Autodesk Inventor part; units mm, degrees
(part 2 of 3)
sketch "Эскиз4" plane through (0, 2, 0) normal (0, 1, 0) x (1, 0, 0)
  arc A0 (90.4395, -37.7453) -> (97.9653, -2.6059) centre (0, 0) ccw construction
  arc A1 (87.1795, -38.3892) -> (90.4395, -37.7453) centre (88.5938, -36.975) ccw construction
  line L0 (87.1795, -38.3892) -> (83.085, -34.2947) construction
  arc A2 (83.085, -34.2947) -> (76.014, -34.2947) centre (79.5495, -37.8302) ccw construction
  line L1 (76.014, -34.2947) -> (67.8823, -42.4264) construction
  line L2 (67.8823, -42.4264) -> (47.1257, -21.6698) construction
  arc A3 (47.1257, -21.6698) -> (46.1335, -19.2746) centre (43.1335, -21.9203) ccw construction
  line L3 (46.1335, -19.2746) -> (46.1335, 19.2746) construction
  arc A4 (46.1335, 19.2746) -> (47.1257, 21.6698) centre (43.1335, 21.9203) ccw construction
  line L4 (47.1257, 21.6698) -> (67.8823, 42.4264) construction
  line L5 (67.8823, 42.4264) -> (76.014, 34.2947) construction
  arc A5 (76.014, 34.2947) -> (83.085, 34.2947) centre (79.5495, 37.8302) ccw construction
  line L6 (83.085, 34.2947) -> (87.1795, 38.3892) construction
  arc A6 (90.4395, 37.7453) -> (87.1795, 38.3892) centre (88.5938, 36.975) ccw construction
  arc A7 (97.9653, 2.6059) -> (90.4395, 37.7453) centre (0, 0) ccw construction
  arc A8 (97.9653, 2.6059) -> (97.9653, -2.6059) centre (101, 0) ccw construction
  circle A9 centre (101, 0) radius 1.9 construction
  arc A10 (93.0503, -48.6481) -> (93.0503, 48.6481) centre (0, 0) ccw construction
  arc A11 (93.0503, 48.6481) -> (88.2704, 49.3795) centre (90.3917, 47.2582) ccw construction
  line L7 (88.2704, 49.3795) -> (85.2064, 46.3155) construction
  arc A12 (73.8927, 46.3155) -> (85.2064, 46.3155) centre (79.5495, 51.9723) ccw construction
  line L8 (73.8927, 46.3155) -> (46.3155, 73.8927) construction
  arc A13 (46.3155, 85.2064) -> (46.3155, 73.8927) centre (51.9723, 79.5495) ccw construction
  line L9 (46.3155, 85.2064) -> (49.3795, 88.2704) construction
  arc A14 (49.3795, 88.2704) -> (48.6481, 93.0503) centre (47.2582, 90.3917) ccw construction
  arc A15 (48.6481, 93.0503) -> (-48.6481, 93.0503) centre (0, 0) ccw construction
  arc A16 (-48.6481, 93.0503) -> (-49.3795, 88.2704) centre (-47.2582, 90.3917) ccw construction
  line L10 (-49.3795, 88.2704) -> (-46.3155, 85.2064) construction
  arc A17 (-46.3155, 73.8927) -> (-46.3155, 85.2064) centre (-51.9723, 79.5495) ccw construction
  line L11 (-46.3155, 73.8927) -> (-73.8927, 46.3155) construction
  arc A18 (-85.2064, 46.3155) -> (-73.8927, 46.3155) centre (-79.5495, 51.9723) ccw construction
  line L12 (-85.2064, 46.3155) -> (-88.2704, 49.3795) construction
  arc A19 (-88.2704, 49.3795) -> (-93.0503, 48.6481) centre (-90.3917, 47.2582) ccw construction
  arc A20 (-93.0503, 48.6481) -> (-93.0503, -48.6481) centre (0, 0) ccw construction
  arc A21 (-93.0503, -48.6481) -> (-88.2704, -49.3795) centre (-90.3917, -47.2582) ccw construction
  line L13 (-88.2704, -49.3795) -> (-85.2064, -46.3155) construction
  arc A22 (-73.8927, -46.3155) -> (-85.2064, -46.3155) centre (-79.5495, -51.9723) ccw construction
  line L14 (-73.8927, -46.3155) -> (-46.3155, -73.8927) construction
  arc A23 (-46.3155, -85.2064) -> (-46.3155, -73.8927) centre (-51.9723, -79.5495) ccw construction
  line L15 (-46.3155, -85.2064) -> (-49.3795, -88.2704) construction
  arc A24 (-49.3795, -88.2704) -> (-48.6481, -93.0503) centre (-47.2582, -90.3917) ccw construction
  arc A25 (-48.6481, -93.0503) -> (-45.42, -94.668) centre (0, 0) ccw construction
  arc A26 (-45.42, -94.668) -> (-43.0355, -94.1655) centre (-44.5548, -92.8648) ccw construction
  line L16 (-43.0355, -94.1655) -> (-18.3802, -65.3664) construction
  arc A27 (-17.477, -64.7643) -> (-18.3802, -65.3664) centre (-16.8609, -66.6671) ccw construction
  line L17 (-17.477, -64.7643) -> (-0.6161, -59.3045) construction
  arc A28 (0.6161, -59.3045) -> (-0.6161, -59.3045) centre (0, -61.2072) ccw construction
  line L18 (0.6161, -59.3045) -> (17.477, -64.7643) construction
  arc A29 (18.3802, -65.3664) -> (17.477, -64.7643) centre (16.8609, -66.6671) ccw construction
  line L19 (18.3802, -65.3664) -> (43.0355, -94.1655) construction
  arc A30 (43.0355, -94.1655) -> (45.42, -94.668) centre (44.5548, -92.8648) ccw construction
  arc A31 (45.42, -94.668) -> (48.6481, -93.0503) centre (0, 0) ccw construction
  arc A32 (48.6481, -93.0503) -> (49.3795, -88.2704) centre (47.2582, -90.3917) ccw construction
  line L20 (49.3795, -88.2704) -> (46.3155, -85.2064) construction
  arc A33 (46.3155, -73.8927) -> (46.3155, -85.2064) centre (51.9723, -79.5495) ccw construction
  line L21 (46.3155, -73.8927) -> (73.8927, -46.3155) construction
  arc A34 (85.2064, -46.3155) -> (73.8927, -46.3155) centre (79.5495, -51.9723) ccw construction
  line L22 (85.2064, -46.3155) -> (88.2704, -49.3795) construction
  arc A35 (88.2704, -49.3795) -> (93.0503, -48.6481) centre (90.3917, -47.2582) ccw construction
  circle A36 centre (-101, 0) radius 1.9 construction
  arc A37 (-90.4395, 37.7453) -> (-97.9653, 2.6059) centre (0, 0) ccw construction
  arc A38 (-87.1795, 38.3892) -> (-90.4395, 37.7453) centre (-88.5938, 36.975) ccw construction
  line L23 (-87.1795, 38.3892) -> (-83.085, 34.2947) construction
  arc A39 (-83.085, 34.2947) -> (-76.014, 34.2947) centre (-79.5495, 37.8302) ccw construction
  line L24 (-76.014, 34.2947) -> (-67.8823, 42.4264) construction
  line L25 (-67.8823, 42.4264) -> (-47.1257, 21.6698) construction
  arc A40 (-47.1257, 21.6698) -> (-46.1335, 19.2746) centre (-43.1335, 21.9203) ccw construction
  line L26 (-46.1335, 19.2746) -> (-46.1335, -19.2746) construction
  arc A41 (-46.1335, -19.2746) -> (-47.1257, -21.6698) centre (-43.1335, -21.9203) ccw construction
  line L27 (-47.1257, -21.6698) -> (-67.8823, -42.4264) construction
  line L28 (-67.8823, -42.4264) -> (-76.014, -34.2947) construction
  arc A42 (-76.014, -34.2947) -> (-83.085, -34.2947) centre (-79.5495, -37.8302) ccw construction
  line L29 (-83.085, -34.2947) -> (-87.1795, -38.3892) construction
  arc A43 (-90.4395, -37.7453) -> (-87.1795, -38.3892) centre (-88.5938, -36.975) ccw construction
  arc A44 (-97.9653, -2.6059) -> (-90.4395, -37.7453) centre (0, 0) ccw construction
  arc A45 (-97.9653, -2.6059) -> (-97.9653, 2.6059) centre (-101, 0) ccw construction
  circle A46 centre (45.1111, -90.3659) radius 2 construction
  circle A47 centre (45.1111, 90.3659) radius 2 construction
  circle A48 centre (90.3659, 45.1111) radius 2 construction
  circle A49 centre (-45.1111, -90.3659) radius 2 construction
  circle A50 centre (90.3659, -45.1111) radius 2 construction
  circle A51 centre (-45.1111, 90.3659) radius 2 construction
  circle A52 centre (-90.3659, 45.1111) radius 2 construction
  circle A53 centre (-90.3659, -45.1111) radius 2 construction
  line L30 (-63.6396, -46.669) -> (-43.8406, -26.8701) construction
  arc A54 (-41.0122, -26.8701) -> (-43.8406, -26.8701) centre (-42.4264, -28.2843) ccw construction
  line L31 (-41.0122, -26.8701) -> (-26.8701, -41.0122) construction
  arc A55 (-26.8701, -43.8406) -> (-26.8701, -41.0122) centre (-28.2843, -42.4264) ccw construction
  line L32 (-26.8701, -43.8406) -> (-46.669, -63.6396) construction
  line L33 (-46.669, -63.6396) -> (-63.6396, -46.669) construction
  line L34 (-42.4264, -67.8823) -> (-21.6698, -47.1257) construction
  arc A56 (-21.6698, -47.1257) -> (-19.2746, -46.1335) centre (-21.9203, -43.1335) ccw construction
  line L35 (-19.2746, -46.1335) -> (19.2746, -46.1335) construction
  arc A57 (19.2746, -46.1335) -> (21.6698, -47.1257) centre (21.9203, -43.1335) ccw construction
  line L36 (21.6698, -47.1257) -> (42.4264, -67.8823) construction
  line L37 (42.4264, -67.8823) -> (37.1244, -73.1843) construction
  arc A58 (34.1909, -73.0707) -> (37.1244, -73.1843) centre (35.7102, -71.7701) ccw construction
  line L38 (34.1909, -73.0707) -> (25.4187, -62.8242) construction
  arc A59 (24.842, -61.8893) -> (25.4187, -62.8242) centre (28.1154, -60.5155) ccw construction
  line L39 (24.842, -61.8893) -> (23.8313, -59.4808) construction
  arc A60 (23.8313, -59.4808) -> (21.0049, -57.3328) centre (20.5578, -60.8546) ccw construction
  line L40 (21.0049, -57.3328) -> (15.1585, -56.5907) construction
  arc A61 (14.5119, -56.4463) -> (15.1585, -56.5907) centre (15.6055, -53.069) ccw construction
  line L41 (14.5119, -56.4463) -> (0.6161, -51.9466) construction
  arc A62 (0.6161, -51.9466) -> (-0.6161, -51.9466) centre (0, -53.8493) ccw construction
  line L42 (-0.6161, -51.9466) -> (-14.5119, -56.4463) construction
  arc A63 (-15.1585, -56.5907) -> (-14.5119, -56.4463) centre (-15.6055, -53.069) ccw construction
  line L43 (-15.1585, -56.5907) -> (-21.0049, -57.3328) construction
  arc A64 (-21.0049, -57.3328) -> (-23.8313, -59.4808) centre (-20.5578, -60.8546) ccw construction
  line L44 (-23.8313, -59.4808) -> (-24.842, -61.8893) construction
  arc A65 (-25.4187, -62.8242) -> (-24.842, -61.8893) centre (-28.1154, -60.5155) ccw construction
  line L45 (-25.4187, -62.8242) -> (-34.1909, -73.0707) construction
  arc A66 (-37.1244, -73.1843) -> (-34.1909, -73.0707) centre (-35.7102, -71.7701) ccw construction
  line L46 (-37.1244, -73.1843) -> (-42.4264, -67.8823) construction
  line L47 (46.669, -63.6396) -> (26.8701, -43.8406) construction
  arc A67 (26.8701, -41.0122) -> (26.8701, -43.8406) centre (28.2843, -42.4264) ccw construction
  line L48 (26.8701, -41.0122) -> (41.0122, -26.8701) construction
  arc A68 (43.8406, -26.8701) -> (41.0122, -26.8701) centre (42.4264, -28.2843) ccw construction
  line L49 (43.8406, -26.8701) -> (63.6396, -46.669) construction
  line L50 (63.6396, -46.669) -> (46.669, -63.6396) construction
  line L51 (63.6396, 46.669) -> (43.8406, 26.8701) construction
  arc A69 (41.0122, 26.8701) -> (43.8406, 26.8701) centre (42.4264, 28.2843) ccw construction
  line L52 (41.0122, 26.8701) -> (26.8701, 41.0122) construction
  arc A70 (26.8701, 43.8406) -> (26.8701, 41.0122) centre (28.2843, 42.4264) ccw construction
  line L53 (26.8701, 43.8406) -> (46.669, 63.6396) construction
  line L54 (46.669, 63.6396) -> (63.6396, 46.669) construction
  line L55 (42.4264, 67.8823) -> (21.6698, 47.1257) construction
  arc A71 (21.6698, 47.1257) -> (19.2746, 46.1335) centre (21.9203, 43.1335) ccw construction
  line L56 (19.2746, 46.1335) -> (-19.2746, 46.1335) construction
  arc A72 (-19.2746, 46.1335) -> (-21.6698, 47.1257) centre (-21.9203, 43.1335) ccw construction
  line L57 (-21.6698, 47.1257) -> (-42.4264, 67.8823) construction
  line L58 (-42.4264, 67.8823) -> (-34.2947, 76.014) construction
  arc A73 (-34.2947, 76.014) -> (-34.2947, 83.085) centre (-37.8302, 79.5495) ccw construction
  line L59 (-34.2947, 83.085) -> (-38.3892, 87.1795) construction
  arc A74 (-37.7453, 90.4395) -> (-38.3892, 87.1795) centre (-36.975, 88.5938) ccw construction
  arc A75 (37.7453, 90.4395) -> (-37.7453, 90.4395) centre (0, 0) ccw construction
  arc A76 (38.3892, 87.1795) -> (37.7453, 90.4395) centre (36.975, 88.5938) ccw construction
  line L60 (38.3892, 87.1795) -> (34.2947, 83.085) construction
  arc A77 (34.2947, 83.085) -> (34.2947, 76.014) centre (37.8302, 79.5495) ccw construction
  line L61 (34.2947, 76.014) -> (42.4264, 67.8823) construction
  line L62 (-19.2746, 40.1335) -> (19.2746, 40.1335) construction
  arc A78 (19.2746, 40.1335) -> (21.6698, 39.1414) centre (21.9203, 43.1335) ccw construction
  line L63 (21.6698, 39.1414) -> (39.1414, 21.6698) construction
  arc A79 (39.1414, 21.6698) -> (40.1335, 19.2746) centre (43.1335, 21.9203) ccw construction
  line L64 (40.1335, 19.2746) -> (40.1335, -19.2746) construction
  arc A80 (40.1335, -19.2746) -> (39.1414, -21.6698) centre (43.1335, -21.9203) ccw construction
  line L65 (39.1414, -21.6698) -> (21.6698, -39.1414) construction
  arc A81 (21.6698, -39.1414) -> (19.2746, -40.1335) centre (21.9203, -43.1335) ccw construction
  line L66 (19.2746, -40.1335) -> (-19.2746, -40.1335) construction
  arc A82 (-19.2746, -40.1335) -> (-21.6698, -39.1414) centre (-21.9203, -43.1335) ccw construction
  line L67 (-21.6698, -39.1414) -> (-39.1414, -21.6698) construction
  arc A83 (-39.1414, -21.6698) -> (-40.1335, -19.2746) centre (-43.1335, -21.9203) ccw construction
  line L68 (-40.1335, -19.2746) -> (-40.1335, 19.2746) construction
  arc A84 (-40.1335, 19.2746) -> (-39.1414, 21.6698) centre (-43.1335, 21.9203) ccw construction
  line L69 (-39.1414, 21.6698) -> (-21.6698, 39.1414) construction
  arc A85 (-21.6698, 39.1414) -> (-19.2746, 40.1335) centre (-21.9203, 43.1335) ccw construction
  circle A86 centre (43.1335, 21.9203) radius 1.6 construction
  circle A87 centre (21.9203, -43.1335) radius 1.6 construction
  circle A88 centre (-21.9203, -43.1335) radius 1.6 construction
  circle A89 centre (-43.1335, -21.9203) radius 1.6 construction
  circle A90 centre (-43.1335, 21.9203) radius 1.6 construction
  circle A91 centre (-21.9203, 43.1335) radius 1.6 construction
  circle A92 centre (43.1335, -21.9203) radius 1.6 construction
  circle A93 centre (21.9203, 43.1335) radius 1.6 construction
  circle A94 centre (-37.8302, 79.5495) radius 1.6 construction
  circle A95 centre (-79.5495, 37.8302) radius 1.6 construction
  circle A96 centre (-79.5495, -37.8302) radius 1.6 construction
  circle A97 centre (79.5495, -37.8302) radius 1.6 construction
  circle A98 centre (37.8302, 79.5495) radius 1.6 construction
  circle A99 centre (79.5495, 37.8302) radius 1.6 construction
  circle A100 centre (-20.5578, -60.8546) radius 1.55 construction
  circle A101 centre (20.5578, -60.8546) radius 1.55 construction
  circle A102 centre (37.8302, -79.5495) radius 1.6 construction
  circle A103 centre (-37.8302, -79.5495) radius 1.6 construction
  line L70 (-46.669, 63.6396) -> (-26.8701, 43.8406) construction
  arc A104 (-26.8701, 41.0122) -> (-26.8701, 43.8406) centre (-28.2843, 42.4264) ccw construction
  line L71 (-26.8701, 41.0122) -> (-41.0122, 26.8701) construction
  arc A105 (-43.8406, 26.8701) -> (-41.0122, 26.8701) centre (-42.4264, 28.2843) ccw construction
  line L72 (-43.8406, 26.8701) -> (-63.6396, 46.669) construction
  line L73 (-63.6396, 46.669) -> (-46.669, 63.6396) construction
  circle A106 centre (0, 0) radius 101 construction
  circle A107 centre (-24, 98.1071) radius 1.6
  circle A108 centre (-24, 98.1071) radius 4
  line L74 (19.2746, 46.1335) -> (-19.2746, 46.1335) construction
  line L75 (0, 46.1335) -> (0, 40.1335) construction
  circle A109 centre (0, 46) radius 1.6
  arc A110 (-3.9978, 46.1335) -> (3.9978, 46.1335) centre (0, 46) ccw construction
  line L76 (-19.2746, 46.1335) -> (-6.2595, 46.1335) construction
  line L77 (6.2595, 46.1335) -> (19.2746, 46.1335) construction
  arc A111 (3.5768, 47.7906) -> (-3.5768, 47.7906) centre (0, 46) ccw
  arc A112 (-6.2595, 46.1335) -> (-3.5768, 47.7906) centre (-6.2595, 49.1335) ccw
  arc A113 (3.5768, 47.7906) -> (6.2595, 46.1335) centre (6.2595, 49.1335) ccw
  line L78 (6.2595, 46.1335) -> (6.2595, 42.1115)
  line L79 (6.2595, 42.1115) -> (-6.2595, 42.1115)
  line L80 (-6.2595, 42.1115) -> (-6.2595, 46.1335)
  line L81 (0, 0) -> (-30.4056, 30.4056) construction
  line L82 (-46.1335, -19.2746) -> (-46.1335, 19.2746) construction
  line L83 (-46.1335, -19.2746) -> (-46.1335, 19.2746) construction
  line L84 (-46.1335, 0) -> (-40.1335, 0) construction
  circle A114 centre (-46, 0) radius 1.6
  arc A115 (-46.1335, -3.9978) -> (-46.1335, 3.9978) centre (-46, 0) ccw construction
  line L85 (-46.1335, 19.2746) -> (-46.1335, 6.2595) construction
  line L86 (-46.1335, -6.2595) -> (-46.1335, -19.2746) construction
  arc A116 (-47.7906, 3.5768) -> (-47.7906, -3.5768) centre (-46, 0) ccw
  arc A117 (-47.7906, 3.5768) -> (-46.1335, 6.2595) centre (-49.1335, 6.2595) ccw
  arc A118 (-46.1335, -6.2595) -> (-47.7906, -3.5768) centre (-49.1335, -6.2595) ccw
  line L87 (-46.1335, -6.2595) -> (-42.1115, -6.2595)
  line L88 (-42.1115, -6.2595) -> (-42.1115, 6.2595)
  line L89 (-42.1115, 6.2595) -> (-46.1335, 6.2595)
  line L90 (0, 0) -> (0, -40.1335) construction
  line L91 (42.1115, 6.2595) -> (46.1335, 6.2595)
  line L92 (42.1115, -6.2595) -> (42.1115, 6.2595)
  arc A119 (46.1335, 6.2595) -> (47.7906, 3.5768) centre (49.1335, 6.2595) ccw
  arc A120 (47.7906, -3.5768) -> (47.7906, 3.5768) centre (46, 0) ccw
  arc A121 (47.7906, -3.5768) -> (46.1335, -6.2595) centre (49.1335, -6.2595) ccw
  line L93 (46.1335, -6.2595) -> (42.1115, -6.2595)
  circle A122 centre (46, 0) radius 1.6
  arc A123 (46.1335, 3.9978) -> (46.1335, -3.9978) centre (46, 0) ccw construction
  circle A124 centre (24, 98.1071) radius 1.6
  circle A125 centre (24, 98.1071) radius 4
  point P0 (46.1335, 0)
  point P1 (0, 101)
  dimension "d89" = 202
  dimension "d90" = 3.2
  dimension "d91" = 8
  dimension "d92" = 3.2
  dimension "d94" = 8
  dimension "d95" = 3
  dimension "d109" = 55
  dimension "d110" = 48
  constraints: 38 end point, 32 point on circle, 29 symmetric about line, 20 centre point, 11 point on line, 6 coincident, 4 midpoint, 4 tangent, 2 perpendicular, 1 collinear, 1 equal radius, 1 vertical, 12 other
  measures "d89" diameter of A106
  measures "d90" diameter of A107
  measures "d91" diameter of A108
  measures "d92" diameter of A109
  measures "d94" diameter of A110
  measures "d95" radius of A112
  measures "d109" distance of A106.end A109.centre
  measures "d110" distance of A124.centre A107.centre
extrude "Выдавливание5" cut sketch "Эскиз4" against normal blind 2 contours A107 | A109 | A114 | A122 | A124
extrude "Выдавливание6" add sketch "Эскиз4" against normal blind 2
sketch "Эскиз5" plane through (0, 2, 0) normal (0, 1, 0) x (1, 0, 0)
  circle A0 centre (-46, 0) radius 1.6 construction
  line L0 (-6.2595, 46.1335) -> (-19.2746, 46.1335) construction
  arc A1 (-19.2746, 46.1335) -> (-21.6698, 47.1257) centre (-21.9203, 43.1335) ccw construction
  line L1 (-21.6698, 47.1257) -> (-42.4264, 67.8823) construction
  line L2 (-42.4264, 67.8823) -> (-34.2947, 76.014) construction
  arc A2 (-34.2947, 76.014) -> (-34.2947, 83.085) centre (-37.8302, 79.5495) ccw construction
  line L3 (-34.2947, 83.085) -> (-38.3892, 87.1795) construction
  arc A3 (-37.7453, 90.4395) -> (-38.3892, 87.1795) centre (-36.975, 88.5938) ccw construction
  arc A4 (-25.8102, 94.5401) -> (-37.7453, 90.4395) centre (0, 0) ccw construction
  arc A5 (-25.8102, 94.5401) -> (-20.7476, 95.7786) centre (-24, 98.1071) ccw construction
  arc A6 (20.7476, 95.7786) -> (-20.7476, 95.7786) centre (0, 0) ccw construction
  arc A7 (38.3892, 87.1795) -> (37.7453, 90.4395) centre (36.975, 88.5938) ccw construction
  line L4 (38.3892, 87.1795) -> (34.2947, 83.085) construction
  arc A8 (34.2947, 83.085) -> (34.2947, 76.014) centre (37.8302, 79.5495) ccw construction
  line L5 (34.2947, 76.014) -> (42.4264, 67.8823) construction
  line L6 (42.4264, 67.8823) -> (21.6698, 47.1257) construction
  arc A9 (21.6698, 47.1257) -> (19.2746, 46.1335) centre (21.9203, 43.1335) ccw construction
  line L7 (19.2746, 46.1335) -> (6.2595, 46.1335) construction
  arc A10 (3.5768, 47.7906) -> (6.2595, 46.1335) centre (6.2595, 49.1335) ccw construction
  arc A11 (3.5768, 47.7906) -> (-3.5768, 47.7906) centre (0, 46) ccw construction
  arc A12 (-6.2595, 46.1335) -> (-3.5768, 47.7906) centre (-6.2595, 49.1335) ccw construction
  circle A13 centre (46, 0) radius 1.6 construction
  arc A14 (48.6481, 93.0503) -> (-48.6481, 93.0503) centre (0, 0) ccw construction
  arc A15 (-48.6481, 93.0503) -> (-49.3795, 88.2704) centre (-47.2582, 90.3917) ccw construction
  line L8 (-49.3795, 88.2704) -> (-46.3155, 85.2064) construction
  arc A16 (-46.3155, 73.8927) -> (-46.3155, 85.2064) centre (-51.9723, 79.5495) ccw construction
  line L9 (-46.3155, 73.8927) -> (-73.8927, 46.3155) construction
  arc A17 (-85.2064, 46.3155) -> (-73.8927, 46.3155) centre (-79.5495, 51.9723) ccw construction
  line L10 (-85.2064, 46.3155) -> (-88.2704, 49.3795) construction
  arc A18 (-88.2704, 49.3795) -> (-93.0503, 48.6481) centre (-90.3917, 47.2582) ccw construction
  arc A19 (-93.0503, 48.6481) -> (-93.0503, -48.6481) centre (0, 0) ccw construction
  arc A20 (-93.0503, -48.6481) -> (-88.2704, -49.3795) centre (-90.3917, -47.2582) ccw construction
  line L11 (-88.2704, -49.3795) -> (-85.2064, -46.3155) construction
  arc A21 (-73.8927, -46.3155) -> (-85.2064, -46.3155) centre (-79.5495, -51.9723) ccw construction
  line L12 (-73.8927, -46.3155) -> (-46.3155, -73.8927) construction
  arc A22 (-46.3155, -85.2064) -> (-46.3155, -73.8927) centre (-51.9723, -79.5495) ccw construction
  line L13 (-46.3155, -85.2064) -> (-49.3795, -88.2704) construction
  arc A23 (-49.3795, -88.2704) -> (-48.6481, -93.0503) centre (-47.2582, -90.3917) ccw construction
  arc A24 (-48.6481, -93.0503) -> (-45.42, -94.668) centre (0, 0) ccw construction
  arc A25 (-45.42, -94.668) -> (-43.0355, -94.1655) centre (-44.5548, -92.8648) ccw construction
  line L14 (-43.0355, -94.1655) -> (-18.3802, -65.3664) construction
  arc A26 (-17.477, -64.7643) -> (-18.3802, -65.3664) centre (-16.8609, -66.6671) ccw construction
  line L15 (-17.477, -64.7643) -> (-0.6161, -59.3045) construction
  arc A27 (0.6161, -59.3045) -> (-0.6161, -59.3045) centre (0, -61.2072) ccw construction
  line L16 (0.6161, -59.3045) -> (17.477, -64.7643) construction
  arc A28 (18.3802, -65.3664) -> (17.477, -64.7643) centre (16.8609, -66.6671) ccw construction
  line L17 (18.3802, -65.3664) -> (43.0355, -94.1655) construction
  arc A29 (43.0355, -94.1655) -> (45.42, -94.668) centre (44.5548, -92.8648) ccw construction
  arc A30 (45.42, -94.668) -> (48.6481, -93.0503) centre (0, 0) ccw construction
  arc A31 (48.6481, -93.0503) -> (49.3795, -88.2704) centre (47.2582, -90.3917) ccw construction
  line L18 (49.3795, -88.2704) -> (46.3155, -85.2064) construction
  arc A32 (46.3155, -73.8927) -> (46.3155, -85.2064) centre (51.9723, -79.5495) ccw construction
  line L19 (46.3155, -73.8927) -> (73.8927, -46.3155) construction
  arc A33 (85.2064, -46.3155) -> (73.8927, -46.3155) centre (79.5495, -51.9723) ccw construction
  line L20 (85.2064, -46.3155) -> (88.2704, -49.3795) construction
  arc A34 (88.2704, -49.3795) -> (93.0503, -48.6481) centre (90.3917, -47.2582) ccw construction
  arc A35 (93.0503, -48.6481) -> (93.0503, 48.6481) centre (0, 0) ccw construction
  arc A36 (93.0503, 48.6481) -> (88.2704, 49.3795) centre (90.3917, 47.2582) ccw construction
  line L21 (88.2704, 49.3795) -> (85.2064, 46.3155) construction
  arc A37 (73.8927, 46.3155) -> (85.2064, 46.3155) centre (79.5495, 51.9723) ccw construction
  line L22 (73.8927, 46.3155) -> (46.3155, 73.8927) construction
  arc A38 (46.3155, 85.2064) -> (46.3155, 73.8927) centre (51.9723, 79.5495) ccw construction
  line L23 (46.3155, 85.2064) -> (49.3795, 88.2704) construction
  arc A39 (49.3795, 88.2704) -> (48.6481, 93.0503) centre (47.2582, 90.3917) ccw construction
  circle A40 centre (-24, 98.1071) radius 1.6 construction
  circle A41 centre (0, 46) radius 1.6 construction
  arc A42 (47.7906, -3.5768) -> (46.1335, -6.2595) centre (49.1335, -6.2595) ccw construction
  arc A43 (47.7906, -3.5768) -> (47.7906, 3.5768) centre (46, 0) ccw construction
  arc A44 (46.1335, 6.2595) -> (47.7906, 3.5768) centre (49.1335, 6.2595) ccw construction
  line L24 (46.1335, 6.2595) -> (46.1335, 19.2746) construction
  arc A45 (46.1335, 19.2746) -> (47.1257, 21.6698) centre (43.1335, 21.9203) ccw construction
  line L25 (47.1257, 21.6698) -> (67.8823, 42.4264) construction
  line L26 (67.8823, 42.4264) -> (76.014, 34.2947) construction
  arc A46 (76.014, 34.2947) -> (83.085, 34.2947) centre (79.5495, 37.8302) ccw construction
  line L27 (83.085, 34.2947) -> (87.1795, 38.3892) construction
  arc A47 (90.4395, 37.7453) -> (87.1795, 38.3892) centre (88.5938, 36.975) ccw construction
  arc A48 (97.9653, 2.6059) -> (90.4395, 37.7453) centre (0, 0) ccw construction
  arc A49 (97.9653, 2.6059) -> (97.9653, -2.6059) centre (101, 0) ccw construction
  arc A50 (90.4395, -37.7453) -> (97.9653, -2.6059) centre (0, 0) ccw construction
  arc A51 (87.1795, -38.3892) -> (90.4395, -37.7453) centre (88.5938, -36.975) ccw construction
  line L28 (87.1795, -38.3892) -> (83.085, -34.2947) construction
  arc A52 (83.085, -34.2947) -> (76.014, -34.2947) centre (79.5495, -37.8302) ccw construction
  line L29 (76.014, -34.2947) -> (67.8823, -42.4264) construction
  line L30 (67.8823, -42.4264) -> (47.1257, -21.6698) construction
  arc A53 (47.1257, -21.6698) -> (46.1335, -19.2746) centre (43.1335, -21.9203) ccw construction
  line L31 (46.1335, -19.2746) -> (46.1335, -6.2595) construction
  circle A54 centre (101, 0) radius 1.9 construction
  circle A55 centre (-101, 0) radius 1.9 construction
  arc A56 (-47.7906, 3.5768) -> (-46.1335, 6.2595) centre (-49.1335, 6.2595) ccw construction
  arc A57 (-47.7906, 3.5768) -> (-47.7906, -3.5768) centre (-46, 0) ccw construction
  arc A58 (-46.1335, -6.2595) -> (-47.7906, -3.5768) centre (-49.1335, -6.2595) ccw construction
  line L32 (-46.1335, -6.2595) -> (-46.1335, -19.2746) construction
  arc A59 (-46.1335, -19.2746) -> (-47.1257, -21.6698) centre (-43.1335, -21.9203) ccw construction
  line L33 (-47.1257, -21.6698) -> (-67.8823, -42.4264) construction
  line L34 (-67.8823, -42.4264) -> (-76.014, -34.2947) construction
  arc A60 (-76.014, -34.2947) -> (-83.085, -34.2947) centre (-79.5495, -37.8302) ccw construction
  line L35 (-83.085, -34.2947) -> (-87.1795, -38.3892) construction
  arc A61 (-90.4395, -37.7453) -> (-87.1795, -38.3892) centre (-88.5938, -36.975) ccw construction
  arc A62 (-97.9653, -2.6059) -> (-90.4395, -37.7453) centre (0, 0) ccw construction
  arc A63 (-97.9653, -2.6059) -> (-97.9653, 2.6059) centre (-101, 0) ccw construction
  arc A64 (-90.4395, 37.7453) -> (-97.9653, 2.6059) centre (0, 0) ccw construction
  arc A65 (-87.1795, 38.3892) -> (-90.4395, 37.7453) centre (-88.5938, 36.975) ccw construction
  line L36 (-87.1795, 38.3892) -> (-83.085, 34.2947) construction
  arc A66 (-83.085, 34.2947) -> (-76.014, 34.2947) centre (-79.5495, 37.8302) ccw construction
  line L37 (-76.014, 34.2947) -> (-67.8823, 42.4264) construction
  line L38 (-67.8823, 42.4264) -> (-47.1257, 21.6698) construction
  arc A67 (-47.1257, 21.6698) -> (-46.1335, 19.2746) centre (-43.1335, 21.9203) ccw construction
  line L39 (-46.1335, 19.2746) -> (-46.1335, 6.2595) construction
  circle A68 centre (45.1111, -90.3659) radius 2 construction
  circle A69 centre (45.1111, 90.3659) radius 2 construction
  circle A70 centre (90.3659, 45.1111) radius 2 construction
  circle A71 centre (-45.1111, -90.3659) radius 2 construction
  circle A72 centre (90.3659, -45.1111) radius 2 construction
  circle A73 centre (-45.1111, 90.3659) radius 2 construction
  circle A74 centre (-90.3659, 45.1111) radius 2 construction
  circle A75 centre (-90.3659, -45.1111) radius 2 construction
  line L40 (-63.6396, -46.669) -> (-43.8406, -26.8701) construction
  arc A76 (-41.0122, -26.8701) -> (-43.8406, -26.8701) centre (-42.4264, -28.2843) ccw construction
  line L41 (-41.0122, -26.8701) -> (-26.8701, -41.0122) construction
  arc A77 (-26.8701, -43.8406) -> (-26.8701, -41.0122) centre (-28.2843, -42.4264) ccw construction
  line L42 (-26.8701, -43.8406) -> (-46.669, -63.6396) construction
  line L43 (-46.669, -63.6396) -> (-63.6396, -46.669) construction
  line L44 (-42.4264, -67.8823) -> (-21.6698, -47.1257) construction
  arc A78 (-21.6698, -47.1257) -> (-19.2746, -46.1335) centre (-21.9203, -43.1335) ccw construction
  line L45 (-19.2746, -46.1335) -> (19.2746, -46.1335) construction
  arc A79 (19.2746, -46.1335) -> (21.6698, -47.1257) centre (21.9203, -43.1335) ccw construction
  line L46 (21.6698, -47.1257) -> (42.4264, -67.8823) construction
  line L47 (42.4264, -67.8823) -> (37.1244, -73.1843) construction
  arc A80 (34.1909, -73.0707) -> (37.1244, -73.1843) centre (35.7102, -71.7701) ccw construction
  line L48 (34.1909, -73.0707) -> (25.4187, -62.8242) construction
  arc A81 (24.842, -61.8893) -> (25.4187, -62.8242) centre (28.1154, -60.5155) ccw construction
  line L49 (24.842, -61.8893) -> (23.8313, -59.4808) construction
  arc A82 (23.8313, -59.4808) -> (21.0049, -57.3328) centre (20.5578, -60.8546) ccw construction
  line L50 (21.0049, -57.3328) -> (15.1585, -56.5907) construction
  arc A83 (14.5119, -56.4463) -> (15.1585, -56.5907) centre (15.6055, -53.069) ccw construction
  line L51 (14.5119, -56.4463) -> (0.6161, -51.9466) construction
  arc A84 (0.6161, -51.9466) -> (-0.6161, -51.9466) centre (0, -53.8493) ccw construction
  line L52 (-0.6161, -51.9466) -> (-14.5119, -56.4463) construction
  arc A85 (-15.1585, -56.5907) -> (-14.5119, -56.4463) centre (-15.6055, -53.069) ccw construction
  line L53 (-15.1585, -56.5907) -> (-21.0049, -57.3328) construction
  arc A86 (-21.0049, -57.3328) -> (-23.8313, -59.4808) centre (-20.5578, -60.8546) ccw construction
  line L54 (-23.8313, -59.4808) -> (-24.842, -61.8893) construction
  arc A87 (-25.4187, -62.8242) -> (-24.842, -61.8893) centre (-28.1154, -60.5155) ccw construction
  line L55 (-25.4187, -62.8242) -> (-34.1909, -73.0707) construction
  arc A88 (-37.1244, -73.1843) -> (-34.1909, -73.0707) centre (-35.7102, -71.7701) ccw construction
  line L56 (-37.1244, -73.1843) -> (-42.4264, -67.8823) construction
  line L57 (46.669, -63.6396) -> (26.8701, -43.8406) construction
  arc A89 (26.8701, -41.0122) -> (26.8701, -43.8406) centre (28.2843, -42.4264) ccw construction
  line L58 (26.8701, -41.0122) -> (41.0122, -26.8701) construction
  arc A90 (43.8406, -26.8701) -> (41.0122, -26.8701) centre (42.4264, -28.2843) ccw construction
  line L59 (43.8406, -26.8701) -> (63.6396, -46.669) construction
  line L60 (63.6396, -46.669) -> (46.669, -63.6396) construction
  line L61 (63.6396, 46.669) -> (43.8406, 26.8701) construction
  arc A91 (41.0122, 26.8701) -> (43.8406, 26.8701) centre (42.4264, 28.2843) ccw construction
  line L62 (41.0122, 26.8701) -> (26.8701, 41.0122) construction
  arc A92 (26.8701, 43.8406) -> (26.8701, 41.0122) centre (28.2843, 42.4264) ccw construction
  line L63 (26.8701, 43.8406) -> (46.669, 63.6396) construction
  line L64 (46.669, 63.6396) -> (63.6396, 46.669) construction
  line L65 (-19.2746, 40.1335) -> (19.2746, 40.1335) construction
  arc A93 (19.2746, 40.1335) -> (21.6698, 39.1414) centre (21.9203, 43.1335) ccw construction
  line L66 (21.6698, 39.1414) -> (39.1414, 21.6698) construction
  arc A94 (39.1414, 21.6698) -> (40.1335, 19.2746) centre (43.1335, 21.9203) ccw construction
  line L67 (40.1335, 19.2746) -> (40.1335, -19.2746) construction
  arc A95 (40.1335, -19.2746) -> (39.1414, -21.6698) centre (43.1335, -21.9203) ccw construction
  line L68 (39.1414, -21.6698) -> (21.6698, -39.1414) construction
  arc A96 (21.6698, -39.1414) -> (19.2746, -40.1335) centre (21.9203, -43.1335) ccw construction
  line L69 (19.2746, -40.1335) -> (-19.2746, -40.1335) construction
  arc A97 (-19.2746, -40.1335) -> (-21.6698, -39.1414) centre (-21.9203, -43.1335) ccw construction
  line L70 (-21.6698, -39.1414) -> (-39.1414, -21.6698) construction
  arc A98 (-39.1414, -21.6698) -> (-40.1335, -19.2746) centre (-43.1335, -21.9203) ccw construction
  line L71 (-40.1335, -19.2746) -> (-40.1335, 19.2746) construction
  arc A99 (-40.1335, 19.2746) -> (-39.1414, 21.6698) centre (-43.1335, 21.9203) ccw construction
  line L72 (-39.1414, 21.6698) -> (-21.6698, 39.1414) construction
  arc A100 (-21.6698, 39.1414) -> (-19.2746, 40.1335) centre (-21.9203, 43.1335) ccw construction
  circle A101 centre (43.1335, 21.9203) radius 1.6 construction
  circle A102 centre (21.9203, -43.1335) radius 1.6 construction
  circle A103 centre (-21.9203, -43.1335) radius 1.6 construction
  circle A104 centre (-43.1335, -21.9203) radius 1.6 construction
  circle A105 centre (-43.1335, 21.9203) radius 1.6 construction
  circle A106 centre (-21.9203, 43.1335) radius 1.6 construction
  circle A107 centre (43.1335, -21.9203) radius 1.6 construction
  circle A108 centre (21.9203, 43.1335) radius 1.6 construction
  circle A109 centre (-37.8302, 79.5495) radius 1.6 construction
  circle A110 centre (-79.5495, 37.8302) radius 1.6 construction
  circle A111 centre (-79.5495, -37.8302) radius 1.6 construction
  circle A112 centre (79.5495, -37.8302) radius 1.6 construction
  circle A113 centre (37.8302, 79.5495) radius 1.6 construction
  circle A114 centre (79.5495, 37.8302) radius 1.6 construction
  circle A115 centre (-20.5578, -60.8546) radius 1.55 construction
  circle A116 centre (20.5578, -60.8546) radius 1.55 construction
  circle A117 centre (37.8302, -79.5495) radius 1.6 construction
  circle A118 centre (-37.8302, -79.5495) radius 1.6 construction
  line L73 (-46.669, 63.6396) -> (-26.8701, 43.8406) construction
  arc A119 (-26.8701, 41.0122) -> (-26.8701, 43.8406) centre (-28.2843, 42.4264) ccw construction
  line L74 (-26.8701, 41.0122) -> (-41.0122, 26.8701) construction
  arc A120 (-43.8406, 26.8701) -> (-41.0122, 26.8701) centre (-42.4264, 28.2843) ccw construction
  line L75 (-43.8406, 26.8701) -> (-63.6396, 46.669) construction
  line L76 (-63.6396, 46.669) -> (-46.669, 63.6396) construction
  circle A121 centre (0, -40) radius 1.6
  line L77 (0, -40.1335) -> (0, 0) construction
  arc A122 (0, -36) -> (-3.6492, -38.362) centre (0, -40) ccw
  line L78 (19.2746, -40.1335) -> (6.3862, -40.1335) construction
  line L79 (19.2746, -40.1335) -> (-19.2746, -40.1335) construction
  line L80 (-6.3862, -40.1335) -> (-19.2746, -40.1335) construction
  arc A123 (3.6492, -38.362) -> (0, -36) centre (0, -40) ccw
  arc A124 (-3.9978, -40.1335) -> (3.9978, -40.1335) centre (0, -40) ccw construction
  arc A125 (3.6492, -38.362) -> (6.3862, -40.1335) centre (6.3862, -37.1335) ccw
  arc A126 (-6.3862, -40.1335) -> (-3.6492, -38.362) centre (-6.3862, -37.1335) ccw
  line L81 (6.3862, -40.1335) -> (3.8373, -44.953)
  line L82 (3.8373, -44.953) -> (-3.2661, -45.2784)
  line L83 (-3.2661, -45.2784) -> (-6.3862, -40.1335)
  arc A127 (20.7476, 95.7786) -> (25.8102, 94.5401) centre (24, 98.1071) ccw projected
  arc A128 (37.7453, 90.4395) -> (25.8102, 94.5401) centre (0, 0) ccw projected
  dimension "d100" = 3.2
  dimension "d101" = 40
  dimension "d103" = 3
  dimension "d104" = 4
  constraints: 12 end point, 12 point on circle, 6 centre point, 6 point on line, 4 tangent, 1 coincident, 1 collinear, 1 equal radius, 1 midpoint, 1 vertical
  measures "d100" diameter of A121
  measures "d101" distance of point (0, 0) A121.centre
  measures "d103" radius of A125
  measures "d104" radius of A124
extrude "Выдавливание7" add sketch "Эскиз5" against normal blind 2
extrude "Выдавливание8" cut sketch "Эскиз5" against normal blind 2 contours A121